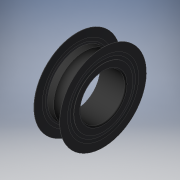
# Autodesk Inventor part: SKF_W 61900 R-2RS1_PART1
Saved by Autodesk Inventor 2019 (Build 230136000, 136)
## iProperties
Created: 2022-08-03
Part Number: SKF_W 61900 R-2RS1_PART1
Material: Generic
Catalog Web Link: www.cadenas.de
Description: -Deep groove ball bearings
Vendor: SKF
Document SubType Name: Modeling
Designer: psAdmin
Manufacturer: SKF
Mass: 11 g
Surface Area: 12.2063 cm^2
Volume: 0.42919 cm^3
Density: 1 g/cm^3
Appearance: PSOLRGB-175-175-175
Category: PARTsolutions
Company: SKF
Title: SKF_W 61900 R-2RS1_PART1
Author: Cadenas PARTsolutions
Comments: Deep groove ball bearings
PSOL_IDENT_0: {$CADENAS_DATA/23d-libs/skf/bearings_units_and_housings/ball_bearings/deep_groove_ball_bearings/bb1_
PSOL_IDENT_1: 001_101.prj},215 {VTYP=3D},{NB=SKF_W 61900 R-2RS1_PART1},{LINA=SKF_W 61900 R-2RS1_PART1},{NN=BB1_001
PSOL_IDENT_2: _101_PART1},{NOPRJ=TRUE},{DATE=29.07.2022 12:16:16},{GEOMDATE=04.07.2022 10:54:51},{VERSION=},{LINEI
PSOL_IDENT_3: D=21610},{WBVAR=},{WBNUMERIC=}  {NB=SKF_W 61900 R-2RS1_PART1},{LINA=SKF_W 61900 R-2RS1_PART1},{KT=DU
PSOL_IDENT_4: MMY},{DESIGNATION=W 61900 R-2RS1},{R12=0.30},{DD=10.000},{D=22.000},{B=6.000},{C=},{CX=},{CXX=1.5},{
PSOL_IDENT_5: CA=1.500},{XXVARIANT=Flanged outer ring},{XXDESIGN=Single row stainless steel},{XXSEALING=Contact se
PSOL_IDENT_6: al on both sides},{DESIGN=dgbbwr2zs},{DESIGNIR=dgbbwr2zs},{VARIANT=Flanged outer ring},{DD1=13.90},{
PSOL_IDENT_7: DD2=13.2},{DD2X=},{DD2A=13.20},{D1=18.20},{D1X=0.00},{D2=19.4},{D2A=19.40},{D3=25},{D3X=},{D3A=25.00
PSOL_IDENT_8: 0},{D4=},{HH=0.000},{BB=0.000},{BBX=},{BBA=0.000},{FF=},{R0MAX=0.000},{R0=0.000},{PITCH=16.00},{DW=3
PSOL_IDENT_9: .175},{DDAMIN=12.000},{DDAMAX=13.000},{DDBMIN=0.000},{DDBMAX=0.000},{DBMIN=0.000},{DAMAX=0.000},{BBA
PSOL_IDENT_10: MIN=0.000},{CAMAX=0.000},{RAMAX=0.300},{LOAD1=2.340},{LOAD2=1.250},{LOAD3=0.054},{SPEED1=0},{SPEED2=
PSOL_IDENT_11: 20000},{KR=0.025},{F0=14.000},{Z=9},{II=1},{MASS=0.011},{BEARING=W 61900 R-2RS1},{RING=},{HELP=1.900
PSOL_IDENT_12: },{HELP2=1.300},{DD1ALG=6.950},{YALG=6.950},{PITCH1=16.000},{DW1=3.175},{YALG1=9.100},{HALG1=1.900},
PSOL_IDENT_13: {SH=6.600},{CU=0.565},{HALG=1.95},{B1=-3.22875},{SHIELDHELP=2},{D4A=0.000},{FFA=0.000},{RS1=},{HELP3=
PSOL_IDENT_14: 0}
NB: SKF_W 61900 R-2RS1_PART1
NT: Deep groove ball bearings
NBSYN: SKF_$DESIGNATION._PART1
LINA: SKF_W 61900 R-2RS1_PART1
CATALOG: SKF
DESIGNATION: W 61900 R-2RS1
R12: 0.3
DD: 10
D: 22
B: 6
XXVARIANT: Flanged outer ring
XXDESIGN: Single row stainless steel
XXSEALING: Contact seal on both sides
DD2: 13.2
D2: 19.4
LOAD1: 2.34
LOAD2: 1.25
LOAD3: 0.054
SPEED1: 0
SPEED2: 20000
BEARING: W 61900 R-2RS1
SUPPLIER: SKF
ARTICLENO: SKF_W 61900 R-2RS1_PART1
BOMINFO: SKF_W 61900 R-2RS1_PART1
CREATOR: CADENAS GmbH
Autodesk Inventor part; units mm, degrees
ref_plane "YZ Plane" through (0, 0, 0) normal (1, 0, 0) x (0, 1, 0)
ref_plane "XZ Plane" through (0, 0, 0) normal (0, 1, 0) x (-1, 0, 0)
ref_plane "XY Plane" through (0, 0, 0) normal (0, 0, 1) x (1, 0, 0)
sketch "Sketch_40" plane through (0, 0, 0) normal (0, 0, 1) x (1, 0, 0)
  line L0 (3, 0) -> (-3, 0)
  line L1 (0, 6.875) -> (0, 5.3)
  arc A0 (0, 5.3) -> (0.3, 5) centre (0.3, 5.3) ccw
  line L2 (0.3, 5) -> (5.7, 5)
  arc A1 (5.7, 5) -> (6, 5.3) centre (5.7, 5.3) ccw
  line L3 (6, 5.3) -> (6, 6.875)
  arc A2 (6, 6.875) -> (5.925, 6.95) centre (5.925, 6.875) ccw
  line L4 (5.925, 6.95) -> (4.1907, 6.95)
  arc A3 (1.8093, 6.95) -> (4.1907, 6.95) centre (3, 8) ccw
  line L5 (1.8093, 6.95) -> (0.075, 6.95)
  arc A4 (0.075, 6.95) -> (0, 6.875) centre (0.075, 6.875) ccw
  constraints: 12 end point, 10 point on circle, 5 centre point
revolve "Revolution1" add sketch "Sketch_40" angle 360 about axis through (3, 0, 0) along (1, 0, 0)
sketch "Sketch_42" plane through (0, 0, 0) normal (0, 0, 1) x (1, 0, 0)
  line L0 (3, 0) -> (-3, 0)
  line L1 (0, 14.6) -> (0, 6.6)
  line L2 (0, 6.6) -> (0.15, 6.6)
  arc A0 (0.15, 6.6) -> (0.45, 6.9) centre (0.15, 6.9) ccw
  line L3 (0.45, 6.9) -> (0.45, 14.3)
  line L4 (0.45, 14.3) -> (5.55, 14.3)
  line L5 (5.55, 14.3) -> (5.55, 6.9)
  arc A1 (5.55, 6.9) -> (5.85, 6.6) centre (5.85, 6.9) ccw
  line L6 (5.85, 6.6) -> (6, 6.6)
  line L7 (6, 6.6) -> (6, 14.6)
  line L8 (6, 14.6) -> (0, 14.6)
  constraints: 18 end point, 4 point on circle, 2 centre point
revolve "Revolution2" cut sketch "Sketch_42" angle 360 about axis through (3, 0, 0) along (1, 0, 0)
sketch "Sketch_44" plane through (0, 0, 0) normal (0, 0, 1) x (1, 0, 0)
  line L0 (5, 0) -> (-5, 0)
  line L1 (5.745, 7.2875) -> (5.835, 6.6)
  line L2 (5.835, 6.6) -> (5.925, 6.6)
  line L3 (5.925, 6.6) -> (5.88, 7.2875)
  line L4 (5.88, 7.2875) -> (5.925, 7.975)
  line L5 (5.925, 7.975) -> (5.925, 9.7)
  line L6 (5.925, 9.7) -> (5.8579, 9.7)
  line L7 (5.8579, 9.7) -> (5.745, 7.975)
  line L8 (5.745, 7.975) -> (5.745, 7.2875)
  constraints: 18 end point
revolve "Revolution3" add sketch "Sketch_44" angle 360 about axis through (5, 0, 0) along (1, 0, 0)
sketch "Sketch_49" plane through (0, 0, 0) normal (0, 0, 1) x (1, 0, 0)
  line L0 (5, 0) -> (-5, 0)
  line L1 (0.105, 6.6) -> (0.195, 6.6)
  line L2 (0.195, 6.6) -> (0.285, 7.2875)
  line L3 (0.285, 7.2875) -> (0.285, 7.975)
  line L4 (0.285, 7.975) -> (0.1721, 9.7)
  line L5 (0.1721, 9.7) -> (0.105, 9.7)
  line L6 (0.105, 9.7) -> (0.105, 7.975)
  line L7 (0.105, 7.975) -> (0.15, 7.2875)
  line L8 (0.15, 7.2875) -> (0.105, 6.6)
  constraints: 18 end point
revolve "Revolution4" add sketch "Sketch_49" angle 360 about axis through (5, 0, 0) along (1, 0, 0)
body "Solid1"
